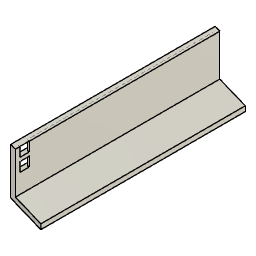
name_sign_LED_holder (Autodesk Fusion 360 design; units mm, degrees)
Autodesk Fusion 360 part; units mm, degrees
sketch "Sketch1" plane through (0, 0, 0) normal (0, 1, 0) x (1, 0, 0)
  line L0 (2.4744, -68.9852) -> (7.4744, -68.9852)
  line L1 (7.4744, -68.9852) -> (7.4744, -22.3387)
  line L2 (7.4744, -22.3387) -> (36.754, -10.3303)
  line L3 (36.754, -10.3303) -> (34.8567, -5.7042)
  line L4 (34.8567, -5.7042) -> (2.4744, -18.9852)
  line L5 (2.4744, -18.9852) -> (2.4744, -68.9852)
  line L6 (2.4744, -68.9852) -> (7.4744, -66.9345)
  line L7 (34.8567, -5.7042) -> (34.8567, -11.1084)
  dimension "d1" = 5
  dimension "d2" = 5
  dimension "d3" = 112.3
  dimension "d16" = 50
  dimension "d18" = 22.3
  dimension "d20" = 35
  constraint horizontal L0
  constraint perpendicular L0 L1
  constraint perpendicular L2 L3
  constraint perpendicular L0 L5
  constraint parallel L2 L4
  constraint coincident L1 L6.end
  constraint parallel L2 L6
  constraint coincident L2 L7.end
  constraint vertical L7
  measures "d1" distance of L0.start L0.end
  measures "d2" distance of L2.end L3.end
  measures "d3" angle of L1 L2
  measures "d16" distance of L0.start L4.end
  measures "d18" angle of L0 L6
  measures "d20" distance of L3.end L4.end
extrude "Extrude1" add sketch "Sketch1" along normal blind 220 contours L1 L2 L4 L5 L6 L7
sketch "Sketch2" plane through (2.4744, 0, 0) normal (-1, 0, 0) x (0, -1, 0)
  line L0 (0, 18.9852) -> (0, 68.9852)
  line L1 (-220, 68.9852) -> (-220, 18.9852)
  line L2 (-220, 18.9852) -> (0, 18.9852)
  line L3 (-215, 66.9852) -> (-5, 66.9852)
  line L4 (-5, 66.9852) -> (-5, 56.9852)
  line L5 (-5, 56.9852) -> (-215, 56.9852)
  line L6 (-215, 56.9852) -> (-215, 66.9852)
  line L7 (-215, 52.9852) -> (-5, 52.9852)
  line L8 (-5, 52.9852) -> (-5, 42.9852)
  line L9 (-5, 42.9852) -> (-215, 42.9852)
  line L10 (-215, 42.9852) -> (-215, 52.9852)
  line L11 (-5, 66.9852) -> (-15, 66.9852)
  line L12 (-15, 56.9852) -> (-5, 56.9852)
  line L13 (-5, 56.9852) -> (-5, 66.9852)
  line L14 (-5, 52.9852) -> (-15, 52.9852)
  line L15 (-15, 42.9852) -> (-5, 42.9852)
  line L16 (-5, 42.9852) -> (-5, 52.9852)
  line L17 (0, 68.9852) -> (-220, 68.9852)
  dimension "d6" = 210
  dimension "d7" = 210
  dimension "d8" = 5
  dimension "d9" = 5
  dimension "d12" = 10
  dimension "d13" = 10
  dimension "d22" = 4
  dimension "d30" = 2
  constraint horizontal L3
  constraint vertical L4
  constraint horizontal L5
  constraint vertical L6
  constraint horizontal L7
  constraint vertical L8
  constraint horizontal L9
  constraint vertical L10
  constraint horizontal L11
  constraint horizontal L12
  constraint vertical L13
  constraint coincident L5 L12.start
  constraint horizontal L14
  constraint horizontal L15
  constraint vertical L16
  constraint coincident L9 L15.start
  measures "d6" distance of L3.start L3.end
  measures "d7" distance of L8.end L9.end
  measures "d8" distance of L1 L6
  measures "d9" distance of L0 L8
  measures "d12" distance of L3.start L5.end
  measures "d13" distance of L7.start L9.end
  measures "d22" distance of L5 L7
  measures "d30" distance of L3 L17
extrude "Extrude2" cut sketch "Sketch2" against normal blind 3 contours L3 L4 L5 L6 L11 L12 L13 | L7 L8 L9 L10 L14 L15 L16
sketch "Sketch3" plane through (5.4744, 0, 0) normal (-1, 0, 0) x (0, -1, 0)
  line L0 (-215, 56.9852) -> (-5, 56.9852)
  line L1 (-5, 56.9852) -> (-5, 66.9852)
  line L2 (-5, 66.9852) -> (-215, 66.9852)
  line L3 (-215, 66.9852) -> (-215, 56.9852)
  line L4 (-5, 66.9852) -> (-15, 66.9852)
  line L5 (-15, 66.9852) -> (-15, 56.9852)
  line L6 (-15, 56.9852) -> (-5, 56.9852)
  line L7 (-5, 56.9852) -> (-5, 66.9852)
  dimension "d33" = 10
  dimension "d34" = 10
  constraint horizontal L4
  constraint vertical L5
  constraint horizontal L6
  constraint vertical L7
  constraint coincident L0 L5.end
  constraint coincident L1.end L2.start
  measures "d33" distance of L1.end L4.end
  measures "d34" distance of L1.end L0.end
sketch "Sketch4" plane through (5.4744, 0, 0) normal (-1, 0, 0) x (0, -1, 0)
  line L0 (-215, 42.9852) -> (-5, 42.9852)
  line L1 (-5, 42.9852) -> (-5, 52.9852)
  line L2 (-215, 52.9852) -> (-215, 42.9852)
  line L3 (-5, 52.9852) -> (-15, 52.9852)
  line L4 (-15, 52.9852) -> (-15, 42.9852)
  line L5 (-15, 42.9852) -> (-5, 42.9852)
  line L6 (-5, 42.9852) -> (-5, 52.9852)
  line L7 (-5, 52.9852) -> (-215, 52.9852)
  dimension "d26" = 10
  dimension "d27" = 10
  constraint horizontal L3
  constraint vertical L4
  constraint horizontal L5
  constraint vertical L6
  constraint coincident L0 L4.end
  constraint coincident L1.end L3.start
  measures "d26" distance of L1.end L3.end
  measures "d27" distance of L1.end L0.end
extrude "Extrude3" cut sketch "Sketch3" sketch "Sketch4" against normal blind 2 contours L0 L1 L2 L4 L5 L6 L7 of sketch 2 contours L0 L1 L3 L4 L5 L6 L7
equation "d4 = 200 mm + 10 mm + 5 mm + 5 mm"
equation "d6 = 200 mm + 10 mm"
equation "d7 = 200 mm + 10 mm"
named bodies: "Name Sign LED Holder"
